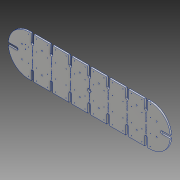
# Autodesk Inventor part: 1311_Former Top_V1
Saved by Autodesk Inventor 2020 (Build 240168000, 168)
## iProperties
Created: 2019-09-11
Part Number: 1311_Former Top_V1
Material: Generic
Document SubType Name: Modeling
Designer: MPI
Density: 1 g/cm^3
Appearance: Aluminum - Flat
Mass: 2918.55 g
Surface Area: 6437.71 cm^2
Volume: 2918.55 cm^3
Author: MPI
Autodesk Inventor part; units mm, degrees
ref_plane "YZ Plane" through (0, 0, 0) normal (1, 0, 0) x (0, 1, 0)
ref_plane "XZ Plane" through (0, 0, 0) normal (0, 1, 0) x (-1, 0, 0)
ref_plane "XY Plane" through (0, 0, 0) normal (0, 0, 1) x (1, 0, 0)
sketch "Sketch1" plane through (0, 0, 0) normal (0, 1, 0) x (-1, 0, 0)
  line L0 (432, 86) -> (-432, 86) construction
  line L1 (-432, -86) -> (432, -86) construction
  arc A0 (432, -86) -> (432, 86) centre (432, 0) ccw construction
  arc A1 (-432, 86) -> (-432, -86) centre (-432, 0) ccw construction
  arc A2 (38, -86) -> (38, -86) centre (0, -86) ccw
  line L2 (-260, -146) -> (-260, -86)
  line L3 (-260, 86) -> (-260, 146)
  line L4 (-280, 146) -> (-280, 86)
  line L5 (-280, -86) -> (-280, -146)
  line L6 (-395, -146) -> (-395, -86)
  line L7 (-415, 146) -> (-415, 86)
  line L8 (-415, -86) -> (-415, -146)
  line L9 (-125, -146) -> (-125, -86)
  line L10 (145, -146) -> (145, -86)
  line L11 (280, -146) -> (280, -86)
  line L12 (280, 86) -> (280, 146)
  line L13 (395, 146) -> (395, 86)
  line L14 (415, -146) -> (415, -86)
  line L15 (415, 86) -> (415, 146)
  line L16 (-577.6571, -10) -> (-518, -10)
  line L17 (518, -10) -> (577.6571, -10)
  line L18 (577.6571, 10) -> (518, 10)
  line L19 (-518, 10) -> (-577.6571, 10)
  arc A3 (-432, 146) -> (-577.6571, 10) centre (-432, 0) ccw
  arc A4 (-577.6571, -10) -> (-432, -146) centre (-432, 0) ccw
  line L20 (-432, -146) -> (-415, -146)
  line L21 (-395, -146) -> (-280, -146)
  line L22 (-280, 146) -> (-395, 146)
  line L23 (-415, 146) -> (-432, 146)
  line L24 (-260, -146) -> (-145, -146)
  line L25 (-145, 146) -> (-260, 146)
  line L26 (-10, 146) -> (-125, 146)
  line L27 (280, -146) -> (395, -146)
  line L28 (415, -146) -> (432, -146)
  line L29 (432, 146) -> (415, 146)
  line L30 (395, 146) -> (280, 146)
  arc A5 (432, -146) -> (577.6571, -10) centre (432, 0) ccw
  arc A6 (577.6571, 10) -> (432, 146) centre (432, 0) ccw
  line L31 (260, 146) -> (145, 146)
  line L32 (125, 146) -> (10, 146)
  line L33 (10, -146) -> (10, -86)
  line L34 (-10, -86) -> (-10, -146)
  line L35 (-125, -146) -> (-10, -146)
  line L36 (10, -146) -> (38.2862, -146)
  line L37 (10, -146) -> (125, -146)
  line L38 (145, -146) -> (260, -146)
  line L39 (260, 146) -> (260, 86)
  line L40 (145, 146) -> (145, 86)
  line L41 (125, 146) -> (125, 86)
  line L42 (10, 146) -> (10, 86)
  line L43 (-10, 146) -> (-10, 86)
  line L44 (-125, 146) -> (-125, 86)
  line L45 (-145, 146) -> (-145, 86)
  line L46 (-395, 146) -> (-395, 86)
  line L47 (395, -146) -> (395, -86)
  line L48 (260, -146) -> (260, -86)
  line L49 (125, -146) -> (125, -86)
  line L50 (-145, -146) -> (-145, -86)
  arc A7 (395, 86) -> (415, 86) centre (405, 86) ccw
  arc A8 (260, 86) -> (280, 86) centre (270, 86) ccw
  arc A9 (125, 86) -> (145, 86) centre (135, 86) ccw
  arc A10 (-145, 86) -> (-125, 86) centre (-135, 86) ccw
  arc A11 (-280, 86) -> (-260, 86) centre (-270, 86) ccw
  arc A12 (-415, 86) -> (-395, 86) centre (-405, 86) ccw
  arc A13 (-518, -10) -> (-518, 10) centre (-518, 0) ccw
  arc A14 (-395, -86) -> (-415, -86) centre (-405, -86) ccw
  arc A15 (-260, -86) -> (-280, -86) centre (-270, -86) ccw
  arc A16 (-125, -86) -> (-145, -86) centre (-135, -86) ccw
  arc A17 (145, -86) -> (125, -86) centre (135, -86) ccw
  arc A18 (280, -86) -> (260, -86) centre (270, -86) ccw
  arc A19 (415, -86) -> (395, -86) centre (405, -86) ccw
  arc A20 (518, 10) -> (518, -10) centre (518, 0) ccw
  arc A21 (10, -86) -> (-10, -86) centre (0, -86) ccw
  arc A22 (-10, 86) -> (10, 86) centre (0, 86) ccw
  point P0 (0, 0)
  point P1 (-517.8487, -10)
  dimension "d0" = 172
  dimension "d1" = 86
  dimension "d2" = 864
  dimension "d3" = 432
  dimension "d113" = 60
  dimension "d117" = 60
  dimension "d122" = 135
  dimension "d125" = 135
  dimension "d129" = 0
  dimension "d130" = 86
  dimension "d131" = 60
  dimension "d132" = 60
  dimension "d133" = 60
  dimension "d134" = 146
  dimension "d137" = 0
  dimension "d178" = 20
  dimension "d179" = 135
  dimension "d181" = 135
  dimension "d182" = 135
  dimension "d183" = 135
  dimension "d185" = 10
  dimension "d242" = 20
  dimension "d243" = 60
  dimension "d244" = 20
  dimension "d245" = 10
  dimension "d246" = 20
  constraints: 98 end point, 82 parallel, 55 point on circle, 37 tangent, 23 centre point, 22 collinear, 14 vertical, 8 horizontal, 7 point on line, 3 equal length, 2 equal radius, 1 coincident, 1 perpendicular, 44 other
  measures "d2" distance of A1.end A0.start
  measures "d3" horizontal distance of A0.start point (0, 0)
  measures "d117" radial gap between concentric circles of A0 A6
  measures "d122" distance between parallel lines of L7 L4
  measures "d125" distance between parallel lines of L15 L12
  measures "d129" distance of A3.centre A1.centre
  measures "d130" radius of A1
  measures "d134" radius of A5
  measures "d137" distance of A3.centre A1.centre
  measures "d178" distance between parallel lines of L43 L42
  measures "d179" distance between parallel lines of L40 L42
  measures "d181" distance between parallel lines of L40 L12
  measures "d182" distance between parallel lines of L45 L43
  measures "d183" distance between parallel lines of L4 L45
  measures "d185" vertical distance of point (0, 0) L18.start
  measures "d242" distance between parallel lines of L47 L14
  measures "d243" distance of L33.start L33.end
  measures "d244" distance between parallel lines of L19 L16
  measures "d245" distance from line of A13.centre L16
  measures "d246" distance between parallel lines of L18 L17
extrude "Extrusion2" add sketch "Sketch1" along normal blind 10 contours A2 L33 A21 L34 | A2 L34 L35 L9 A16 L50 L24 L2 A15 L5 L21 L6 A14 L8 L20 A4 L16 A13 L19 A3 L23 L7 A12 L46 L22 L4 A11 L3 L25 L45 A10 L44 L26 L43 A22 L42 L32 L41 A9 L40 L31 L39 A8 L12 L30 L13 A7 L15 L29 A6 L18 A20 L17 A5 L28 L14 A19 L47 L27 L11 A18 L48 L38 L10 A17 L49 L37 L36 L33 picked at (-12.6123, -109.4048)
sketch "Sketch2" plane through (0, 0, 0) normal (0, -1, 0) x (1, 0, 0)
  circle A0 centre (-480, 48) radius 4
  circle A1 centre (-480, -48) radius 4
  circle A2 centre (-337.5, 76) radius 4
  circle A3 centre (-337.5, -76) radius 4
  circle A4 centre (337.5, 76) radius 4
  circle A5 centre (337.5, -76) radius 4
  circle A6 centre (480, 48) radius 4
  circle A7 centre (480, -48) radius 4
  circle A8 centre (0, 0) radius 13
  circle A9 centre (67.5, -76) radius 4
  circle A10 centre (-67.5, -76) radius 4
  circle A11 centre (-67.5, 76) radius 4
  circle A12 centre (67.5, 76) radius 4
  line L0 (395, -86) -> (395, -146) projected
  line L1 (395, 146) -> (395, 86) projected
  line L2 (125, -86) -> (125, -146) projected
  line L3 (125, 146) -> (125, 86) projected
  line L4 (-125, -146) -> (-125, -86) projected
  line L5 (-125, 86) -> (-125, 146) projected
  line L6 (-280, -86) -> (-280, -146) projected
  line L7 (-280, 146) -> (-280, 86) projected
  point P0 (-518, 0)
  point P1 (518, 0)
  dimension "d43" = 76
  dimension "d44" = 76
  dimension "d45" = 76
  dimension "d46" = 76
  dimension "d51" = 8
  dimension "d63" = 26
  dimension "d138" = 38
  dimension "d139" = 48
  dimension "d140" = 48
  dimension "d141" = 38
  dimension "d142" = 38
  dimension "d143" = 48
  dimension "d144" = 48
  dimension "d145" = 38
  dimension "d166" = 960
  dimension "d167" = 76
  dimension "d168" = 76
  dimension "d169" = 76
  dimension "d170" = 76
  dimension "d232" = 57.5
  dimension "d233" = 57.5
  dimension "d234" = 57.5
  dimension "d235" = 57.5
  dimension "d236" = 57.5
  dimension "d237" = 57.5
  dimension "d238" = 57.5
  dimension "d239" = 57.5
  constraints: 13 centre point, 11 equal radius, 1 coincident
  measures "d43" vertical distance of point (0, 0) A2.centre
  measures "d44" vertical distance of point (0, 0) A3.centre
  measures "d45" vertical distance of A4.centre point (0, 0)
  measures "d46" vertical distance of point (0, 0) A5.centre
  measures "d51" diameter of A0
  measures "d63" diameter of A8
  measures "d138" horizontal distance of point (-518, 0) A0.centre
  measures "d139" vertical distance of point (-518, 0) A0.centre
  measures "d140" vertical distance of A1.centre point (-518, 0)
  measures "d141" horizontal distance of point (-518, 0) A1.centre
  measures "d142" horizontal distance of point (518, 0) A6.centre
  measures "d143" vertical distance of point (518, 0) A6.centre
  measures "d144" vertical distance of A7.centre point (518, 0)
  measures "d145" horizontal distance of point (518, 0) A7.centre
  measures "d166" distance of A1.centre A7.centre
  measures "d167" vertical distance of point (0, 0) A10.centre
  measures "d168" vertical distance of A11.centre point (0, 0)
  measures "d169" vertical distance of point (0, 0) A9.centre
  measures "d170" vertical distance of point (0, 0) A12.centre
  measures "d232" distance from line of A5.centre L0
  measures "d233" distance from line of L1 A4.centre
  measures "d234" distance from line of A9.centre L2
  measures "d235" distance from line of L3 A12.centre
  measures "d236" distance from line of L4 A10.centre
  measures "d237" distance from line of A11.centre L5
  measures "d238" distance from line of A3.centre L6
  measures "d239" distance from line of L7 A2.centre
extrude "Extrusion3" cut sketch "Sketch2" against normal blind 260
sketch "Sketch9" plane through (0, 10, 0) normal (0, 1, 0) x (1, 0, 0)
  circle A0 centre (-405, 66) radius 2
  circle A1 centre (0, 0) radius 13 projected
  line L0 (0, 0) -> (0, 116) construction
  line L1 (10, 146) -> (10, 86) projected
  arc A2 (-415, 86) -> (-395, 86) centre (-405, 86) ccw projected
  circle A3 centre (-405, 59) radius 2
  circle A4 centre (-405, 52) radius 2
  circle A5 centre (-405, 45) radius 2
  circle A6 centre (-405, 38) radius 2
  circle A7 centre (-405, 31) radius 2
  circle A8 centre (-405, 24) radius 2
  circle A9 centre (-405, 17) radius 2
  circle A10 centre (-405, 10) radius 2
  arc A11 (-280, 86) -> (-260, 86) centre (-270, 86) ccw projected
  arc A12 (-260, -86) -> (-280, -86) centre (-270, -86) ccw projected
  line L2 (-270, 86) -> (-270, -86) construction
  arc A13 (-145, 86) -> (-125, 86) centre (-135, 86) ccw projected
  arc A14 (-125, -86) -> (-145, -86) centre (-135, -86) ccw projected
  line L3 (-135, 86) -> (-135, -86) construction
  arc A15 (-10, 86) -> (10, 86) centre (0, 86) ccw projected
  arc A16 (10, -86) -> (-10, -86) centre (0, -86) ccw projected
  line L4 (0, 86) -> (0, -86) construction
  arc A17 (125, 86) -> (145, 86) centre (135, 86) ccw projected
  arc A18 (145, -86) -> (125, -86) centre (135, -86) ccw projected
  line L5 (135, 86) -> (135, -86) construction
  arc A19 (260, 86) -> (280, 86) centre (270, 86) ccw projected
  arc A20 (280, -86) -> (260, -86) centre (270, -86) ccw projected
  line L6 (270, 86) -> (270, -86) construction
  arc A21 (395, 86) -> (415, 86) centre (405, 86) ccw projected
  arc A22 (415, -86) -> (395, -86) centre (405, -86) ccw projected
  line L7 (405, 86) -> (405, -86) construction
  circle A23 centre (-270, 66) radius 2
  circle A24 centre (-270, 59) radius 2
  circle A25 centre (-270, 52) radius 2
  circle A26 centre (-270, 45) radius 2
  circle A27 centre (-270, 38) radius 2
  circle A28 centre (-270, 31) radius 2
  circle A29 centre (-270, 24) radius 2
  circle A30 centre (-270, 17) radius 2
  circle A31 centre (-270, 10) radius 2
  circle A32 centre (-135, 66) radius 2
  circle A33 centre (-135, 59) radius 2
  circle A34 centre (-135, 52) radius 2
  circle A35 centre (-135, 45) radius 2
  circle A36 centre (-135, 38) radius 2
  circle A37 centre (-135, 31) radius 2
  circle A38 centre (-135, 24) radius 2
  circle A39 centre (-135, 17) radius 2
  circle A40 centre (-135, 10) radius 2
  circle A41 centre (0, 66) radius 2
  circle A42 centre (0, 59) radius 2
  circle A43 centre (0, 52) radius 2
  circle A44 centre (0, 45) radius 2
  circle A45 centre (0, 38) radius 2
  circle A46 centre (0, 31) radius 2
  circle A47 centre (0, 24) radius 2
  circle A48 centre (0, 17) radius 2
  circle A49 centre (0, 10) radius 2
  circle A50 centre (135, 66) radius 2
  circle A51 centre (135, 59) radius 2
  circle A52 centre (135, 52) radius 2
  circle A53 centre (135, 45) radius 2
  circle A54 centre (135, 38) radius 2
  circle A55 centre (135, 31) radius 2
  circle A56 centre (135, 24) radius 2
  circle A57 centre (135, 17) radius 2
  circle A58 centre (135, 10) radius 2
  circle A59 centre (270, 66) radius 2
  circle A60 centre (270, 59) radius 2
  circle A61 centre (270, 52) radius 2
  circle A62 centre (270, 45) radius 2
  circle A63 centre (270, 38) radius 2
  circle A64 centre (270, 31) radius 2
  circle A65 centre (270, 24) radius 2
  circle A66 centre (270, 17) radius 2
  circle A67 centre (270, 10) radius 2
  circle A68 centre (405, 66) radius 2
  circle A69 centre (405, 59) radius 2
  circle A70 centre (405, 52) radius 2
  circle A71 centre (405, 45) radius 2
  circle A72 centre (405, 38) radius 2
  circle A73 centre (405, 31) radius 2
  circle A74 centre (405, 24) radius 2
  circle A75 centre (405, 17) radius 2
  circle A76 centre (405, 10) radius 2
  arc A77 (-518, -10) -> (-518, 10) centre (-518, 0) ccw projected
  line L8 (-518, 0) -> (674.2682, 0) construction
  circle A78 centre (-405, -66) radius 2
  circle A79 centre (-405, -59) radius 2
  circle A80 centre (-405, -52) radius 2
  circle A81 centre (-405, -45) radius 2
  circle A82 centre (-405, -38) radius 2
  circle A83 centre (-405, -31) radius 2
  circle A84 centre (-405, -24) radius 2
  circle A85 centre (-405, -17) radius 2
  circle A86 centre (-405, -10) radius 2
  line L9 (270, -86) -> (270, 86) construction
  line L10 (405, -86) -> (405, 86) construction
  circle A87 centre (-270, -66) radius 2
  circle A88 centre (-270, -59) radius 2
  circle A89 centre (-270, -10) radius 2
  circle A90 centre (-270, -17) radius 2
  circle A91 centre (-270, -24) radius 2
  circle A92 centre (-270, -31) radius 2
  circle A93 centre (-270, -38) radius 2
  circle A94 centre (-270, -45) radius 2
  circle A95 centre (-270, -52) radius 2
  circle A96 centre (-135, -66) radius 2
  circle A97 centre (-135, -59) radius 2
  circle A98 centre (-135, -10) radius 2
  circle A99 centre (-135, -17) radius 2
  circle A100 centre (-135, -24) radius 2
  circle A101 centre (-135, -31) radius 2
  circle A102 centre (-135, -38) radius 2
  circle A103 centre (-135, -45) radius 2
  circle A104 centre (-135, -52) radius 2
  circle A105 centre (0, -66) radius 2
  circle A106 centre (0, -59) radius 2
  circle A107 centre (0, -10) radius 2
  circle A108 centre (0, -17) radius 2
  circle A109 centre (0, -24) radius 2
  circle A110 centre (0, -31) radius 2
  circle A111 centre (0, -38) radius 2
  circle A112 centre (0, -45) radius 2
  circle A113 centre (0, -52) radius 2
  circle A114 centre (135, -66) radius 2
  circle A115 centre (135, -59) radius 2
  circle A116 centre (135, -10) radius 2
  circle A117 centre (135, -17) radius 2
  circle A118 centre (135, -24) radius 2
  circle A119 centre (135, -31) radius 2
  circle A120 centre (135, -38) radius 2
  circle A121 centre (135, -45) radius 2
  circle A122 centre (135, -52) radius 2
  circle A123 centre (270, -66) radius 2
  circle A124 centre (270, -59) radius 2
  circle A125 centre (270, -10) radius 2
  circle A126 centre (270, -17) radius 2
  circle A127 centre (270, -24) radius 2
  circle A128 centre (270, -31) radius 2
  circle A129 centre (270, -38) radius 2
  circle A130 centre (270, -45) radius 2
  circle A131 centre (270, -52) radius 2
  circle A132 centre (405, -66) radius 2
  circle A133 centre (405, -59) radius 2
  circle A134 centre (405, -10) radius 2
  circle A135 centre (405, -17) radius 2
  circle A136 centre (405, -24) radius 2
  circle A137 centre (405, -31) radius 2
  circle A138 centre (405, -38) radius 2
  circle A139 centre (405, -45) radius 2
  circle A140 centre (405, -52) radius 2
  dimension "d196" = 4
  dimension "d199" = 7
  dimension "d204" = 20
  dimension "d207" = 7
  dimension "d227" = 7
  dimension "d326" = 4
  dimension "d327" = 7
  dimension "d328" = 7
  dimension "d329" = 7
  dimension "d342" = 4
  dimension "d343" = 7
  dimension "d344" = 7
  dimension "d345" = 7
  dimension "d358" = 4
  dimension "d359" = 7
  dimension "d360" = 7
  dimension "d361" = 7
  dimension "d374" = 4
  dimension "d375" = 7
  dimension "d376" = 7
  dimension "d377" = 7
  dimension "d390" = 4
  dimension "d391" = 7
  dimension "d392" = 7
  dimension "d393" = 7
  dimension "d406" = 4
  dimension "d407" = 7
  dimension "d408" = 7
  dimension "d409" = 7
  constraints: 126 centre point, 74 symmetric about line, 20 end point, 9 vertical, 1 horizontal, 1 parallel, 80 other
  measures "d196" diameter of A0
  measures "d199" distance of A0.centre point (-405, 59)
  measures "d204" distance of A0.centre A2.centre
  measures "d207" distance of A0.centre A3.centre
  measures "d227" distance of A9.centre A10.centre
  measures "d326" diameter of A23
  measures "d327" distance of A23.centre point (-270, 59)
  measures "d328" distance of A23.centre A24.centre
  measures "d329" distance of A30.centre A31.centre
  measures "d342" diameter of A32
  measures "d343" distance of A32.centre point (-135, 59)
  measures "d344" distance of A32.centre A33.centre
  measures "d345" distance of A39.centre A40.centre
  measures "d358" diameter of A41
  measures "d359" distance of A41.centre point (0, 59)
  measures "d360" distance of A41.centre A42.centre
  measures "d361" distance of A48.centre A49.centre
  measures "d374" diameter of A50
  measures "d375" distance of A50.centre point (135, 59)
  measures "d376" distance of A50.centre A51.centre
  measures "d377" distance of A57.centre A58.centre
  measures "d390" diameter of A59
  measures "d391" distance of A59.centre point (270, 59)
  measures "d392" distance of A59.centre A60.centre
  measures "d393" distance of A66.centre A67.centre
  measures "d406" diameter of A68
  measures "d407" distance of A68.centre point (405, 59)
  measures "d408" distance of A68.centre A69.centre
  measures "d409" distance of A75.centre A76.centre
extrude "Extrusion9" cut sketch "Sketch9" against normal through all contours A0 | A3 | A4 | A5 | A6 | A7 | A8 | A9 | A10 | A23 | A24 | A25 | A26 | A27 | A28 | A29 | A30 | A31 | A32 | A33 | A34 | A35 | A36 | A37 | A38 | A39 | A40 | A41 | A42 | A43 | A44 | A45 | A46 | A47 | A48 | A49 | A50 | A51 | A52 | A53 | A54 | A55 | A56 | A57 | A58 | A59 | A60 | A61 | A62 | A63 | A64 | A65 | A66 | A67 | A68 | A69 | A70 | A71 | A72 | A73 | A74 | A75 | A76 | A78 | A79 | A80 | A81 | A82 | A83 | A84 | A85 | A86 | A87 | A88 | A89 | A90 | A91 | A92 | A93 | A94 | A95 | A96 | A97 | A98 | A99 | A100 | A101 | A102 | A103 | A104 | A105 | A106 | A107 | A108 | A109 | A110 | A111 | A112 | A113 | A114 | A115 | A116 | A117 | A118 | A119 | A120 | A121 | A122 | A123 | A124 | A125 | A126 | A127 | A128 | A129 | A130 | A131 | A132 | A133 | A134 | A135 | A136 | A137 | A138 | A139 | A140
sketch "Sketch11" plane through (0, 10, 0) normal (0, 1, 0) x (1, 0, 0)
  line L0 (-395, 146) -> (-395, 86) projected
  line L1 (-280, 146) -> (-395, 146) projected
  circle A0 centre (-435, 130) radius 1.9
  circle A1 centre (-435, 50) radius 1.9
  circle A2 centre (-435, -50) radius 1.9
  circle A3 centre (-435, -130) radius 1.9
  circle A4 centre (-375, 130) radius 1.9
  circle A5 centre (-375, 50) radius 1.9
  circle A6 centre (-375, -50) radius 1.9
  circle A7 centre (-375, -130) radius 1.9
  line L2 (-435, 130) -> (716.3943, 130) construction
  line L3 (-435, 50) -> (733.336, 50) construction
  line L4 (-435, -50) -> (716.3943, -50) construction
  line L5 (-435, -130) -> (678.9235, -130) construction
  line L6 (-375, 176.56) -> (-375, -200.787) construction
  line L7 (-435, 166.5955) -> (-435, -182.2247) construction
  line L8 (-415, -146) -> (-415, -86) projected
  circle A8 centre (-300, 130) radius 1.9
  circle A9 centre (-300, 50) radius 1.9
  circle A10 centre (-300, -50) radius 1.9
  circle A11 centre (-300, -130) radius 1.9
  circle A12 centre (-240, 130) radius 1.9
  circle A13 centre (-240, 50) radius 1.9
  circle A14 centre (-240, -50) radius 1.9
  circle A15 centre (-240, -130) radius 1.9
  line L9 (-240, 176.56) -> (-240, -200.787) construction
  line L10 (-300, 166.5955) -> (-300, -182.2247) construction
  circle A16 centre (-165, 130) radius 1.9
  circle A17 centre (-165, 50) radius 1.9
  circle A18 centre (-165, -50) radius 1.9
  circle A19 centre (-165, -130) radius 1.9
  circle A20 centre (-105, 130) radius 1.9
  circle A21 centre (-105, 50) radius 1.9
  circle A22 centre (-105, -50) radius 1.9
  circle A23 centre (-105, -130) radius 1.9
  line L11 (-105, 176.56) -> (-105, -200.787) construction
  line L12 (-165, 166.5955) -> (-165, -182.2247) construction
  circle A24 centre (-30, 130) radius 1.9
  circle A25 centre (-30, 50) radius 1.9
  circle A26 centre (-30, -50) radius 1.9
  circle A27 centre (-30, -130) radius 1.9
  circle A28 centre (30, 130) radius 1.9
  circle A29 centre (30, 50) radius 1.9
  circle A30 centre (30, -50) radius 1.9
  circle A31 centre (30, -130) radius 1.9
  line L13 (30, 176.56) -> (30, -200.787) construction
  line L14 (-30, 166.5955) -> (-30, -182.2247) construction
  circle A32 centre (105, 130) radius 1.9
  circle A33 centre (105, 50) radius 1.9
  circle A34 centre (105, -50) radius 1.9
  circle A35 centre (105, -130) radius 1.9
  circle A36 centre (165, 130) radius 1.9
  circle A37 centre (165, 50) radius 1.9
  circle A38 centre (165, -50) radius 1.9
  circle A39 centre (165, -130) radius 1.9
  line L15 (165, 176.56) -> (165, -200.787) construction
  line L16 (105, 166.5955) -> (105, -182.2247) construction
  circle A40 centre (240, 130) radius 1.9
  circle A41 centre (240, 50) radius 1.9
  circle A42 centre (240, -50) radius 1.9
  circle A43 centre (240, -130) radius 1.9
  circle A44 centre (300, 130) radius 1.9
  circle A45 centre (300, 50) radius 1.9
  circle A46 centre (300, -50) radius 1.9
  circle A47 centre (300, -130) radius 1.9
  line L17 (300, 176.56) -> (300, -200.787) construction
  line L18 (240, 166.5955) -> (240, -182.2247) construction
  circle A48 centre (375, 130) radius 1.9
  circle A49 centre (375, 50) radius 1.9
  circle A50 centre (375, -50) radius 1.9
  circle A51 centre (375, -130) radius 1.9
  circle A52 centre (435, 130) radius 1.9
  circle A53 centre (435, 50) radius 1.9
  circle A54 centre (435, -50) radius 1.9
  circle A55 centre (435, -130) radius 1.9
  line L19 (435, 176.56) -> (435, -200.787) construction
  line L20 (375, 166.5955) -> (375, -182.2247) construction
  line L21 (-280, 86) -> (-280, 146) projected
  line L22 (-145, 86) -> (-145, 146) projected
  line L23 (-125, 146) -> (-125, 86) projected
  line L24 (-260, 146) -> (-260, 86) projected
  line L25 (-10, 86) -> (-10, 146) projected
  line L26 (10, 146) -> (10, 86) projected
  line L27 (125, 86) -> (125, 146) projected
  line L28 (145, 146) -> (145, 86) projected
  line L29 (260, 86) -> (260, 146) projected
  line L30 (280, 146) -> (280, 86) projected
  line L31 (395, 86) -> (395, 146) projected
  line L32 (415, 146) -> (415, 86) projected
  point P0 (0, 0)
  dimension "d250" = 3.8
  dimension "d260" = 20
  dimension "d261" = 20
  dimension "d264" = 3.8
  dimension "d265" = 3.8
  dimension "d266" = 3.8
  dimension "d267" = 3.8
  dimension "d268" = 3.8
  dimension "d269" = 3.8
  dimension "d270" = 20
  dimension "d271" = 20
  dimension "d272" = 20
  dimension "d273" = 20
  dimension "d274" = 20
  dimension "d275" = 20
  dimension "d276" = 20
  dimension "d277" = 20
  dimension "d278" = 20
  dimension "d279" = 20
  dimension "d280" = 20
  dimension "d281" = 20
  constraints: 60 point on line, 56 centre point, 49 equal radius, 36 end point, 14 vertical, 4 horizontal
  measures "d250" diameter of A0
  measures "d260" distance between parallel lines of L6 L0
  measures "d261" distance between parallel lines of L8 L7
  measures "d264" diameter of A8
  measures "d265" diameter of A16
  measures "d266" diameter of A24
  measures "d267" diameter of A32
  measures "d268" diameter of A40
  measures "d269" diameter of A48
  measures "d270" distance between parallel lines of L21 L10
  measures "d271" distance between parallel lines of L22 L12
  measures "d272" distance between parallel lines of L11 L23
  measures "d273" distance between parallel lines of L24 L9
  measures "d274" distance between parallel lines of L25 L14
  measures "d275" distance between parallel lines of L26 L13
  measures "d276" distance between parallel lines of L27 L16
  measures "d277" distance between parallel lines of L28 L15
  measures "d278" distance between parallel lines of L29 L18
  measures "d279" distance between parallel lines of L30 L17
  measures "d280" distance between parallel lines of L31 L20
  measures "d281" distance between parallel lines of L32 L19
extrude "Extrusion10" cut sketch "Sketch11" against normal through all
sketch "Sketch12" plane through (0, 0, 0) normal (0, -1, 0) x (1, 0, 0)
  circle A0 centre (-480, 48) radius 4 projected
  circle A1 centre (-455.5, 26) radius 2.555
  circle A2 centre (-455.5, 56) radius 2.555
  line L0 (-415, 146) -> (-415, 86) projected
  arc A3 (-415, 86) -> (-395, 86) centre (-405, 86) ccw projected
  point P0 (0, 0)
  dimension "d416" = 5.11
  dimension "d417" = 5.11
  dimension "d419" = 30
  dimension "d420" = 40.5
  dimension "d421" = 30
  constraints: 2 centre point
  measures "d416" diameter of A1
  measures "d417" diameter of A2
  measures "d419" distance of A1.centre A2.centre
  measures "d420" distance from line of L0 A2.centre
  measures "d421" vertical distance of A3.centre A2.centre
extrude "Extrusion11" cut sketch "Sketch12" against normal through all contours A1 | A2
equation "\"d52\" = d47"
equation "\"d47\" = 260"
body "Solid2"
